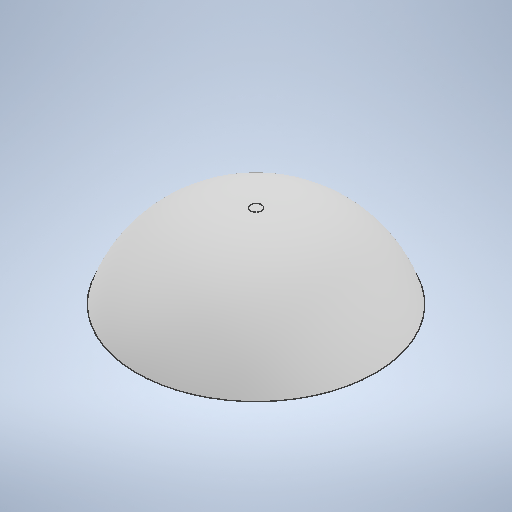
# Autodesk Inventor part: nob_L
Saved by Autodesk Inventor 2025 (Build 290162000, 162)
## iProperties
Created: 2026-02-25
Part Number: nob_L
Material: 一般
Document SubType Name: Modeling
Designer: sooo1
Density: 1 g/cm^3
Appearance: 既定
Author: sooo1
Autodesk Inventor part; units mm, degrees
ref_plane "YZ Plane" through (0, 0, 0) normal (1, 0, 0) x (0, 1, 0)
ref_plane "XZ Plane" through (0, 0, 0) normal (0, 1, 0) x (-1, 0, 0)
ref_plane "XY Plane" through (0, 0, 0) normal (0, 0, 1) x (1, 0, 0)
sketch "スケッチ1" plane through (0, 0, 0) normal (0, 0, 1) x (1, 0, 0)
  line L0 (2, 8) -> (-2, 8) construction
  line L1 (2, 8) -> (2, 13.5) construction
  line L2 (-2, 13.5) -> (2, 13.5) construction
  line L3 (-2, 8) -> (-2, 13.5) construction
  line L4 (-10, 8) -> (10, 8)
  line L5 (10, 8) -> (10, 18)
  line L6 (10, 18) -> (-10, 18)
  line L7 (-10, 18) -> (-10, 8)
  line L8 (0, -3.6) -> (0, 21.6) construction
  line L9 (-2.3, 13.8) -> (-2.3, 8)
  line L10 (-2.3, 13.8) -> (2.3, 13.8)
  line L11 (2.3, 13.8) -> (2.3, 8)
  line L12 (-10, 11) -> (10, 11)
  line L13 (-10, 14.5) -> (10, 14.5) construction
  point P0 (0, 0)
  point P1 (0, 18)
  point P2 (-2.3, 11)
  point P3 (2.3, 11)
  dimension "d0" = 20
  dimension "d1" = 10
  dimension "d2" = 0.3
  dimension "d3" = 0.3
  dimension "d4" = 0.3
  dimension "d5" = 3
  dimension "d6" = 3.5
  constraints: 18 end point, 7 point on line, 5 perpendicular, 2 horizontal, 2 parallel, 1 collinear, 1 midpoint
  measures "d0" distance of L5.end L6.end
  measures "d1" distance of L4.end L5.end
  measures "d2" distance between parallel lines of L2 L10
  measures "d3" distance between parallel lines of L9 L3
  measures "d4" distance between parallel lines of L1 L11
  measures "d5" distance between parallel lines of L4 L12
  measures "d6" distance between parallel lines of L12 L13
extrude "押し出し1" add sketch "スケッチ1" along normal mid plane 20 contours L7 L6 L5 L12 L11 L10 L9 | L9 L10 L11 L12
extrude "押し出し2" cut sketch "スケッチ1" along normal mid plane 2.2 contours L9 L10 L11 L12
fillet "フィレット1" radius 10 4 edges at (-10, 14.5, 10) (-10, 14.5, -10) (10, 14.5, -10) (10, 14.5, 10)
fillet "フィレット2" radius 10 3 edges at (0, 18, 10) (-7.0711, 18, 7.0711) (-10, 18, 0)
